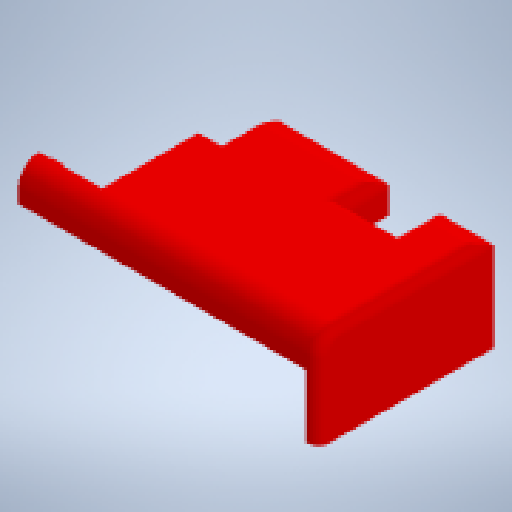
# Autodesk Inventor part: hand_finger_cover
Saved by Autodesk Inventor 2024.1 (Build 281209000, 209)
## iProperties
Created: 2025-03-27
Part Number: hand_finger_cover
Material: 一般
Document SubType Name: Modeling
Designer: hibik
Density: 1 g/cm^3
Appearance: 既定
Author: hibik
Autodesk Inventor part; units mm, degrees
ref_plane "YZ Plane" through (0, 0, 0) normal (1, 0, 0) x (0, 1, 0)
ref_plane "XZ Plane" through (0, 0, 0) normal (0, 1, 0) x (-1, 0, 0)
ref_plane "XY Plane" through (0, 0, 0) normal (0, 0, 1) x (1, 0, 0)
sketch "スケッチ1" plane through (0, 0, 0) normal (1, 0, 0) x (0, 1, 0)
  line L0 (0, 0) -> (22.8, 0)
  line L1 (22.8, 0) -> (22.8, 41.3)
  line L2 (22.8, 41.3) -> (0, 41.3)
  line L3 (0, 41.3) -> (0, 0)
  arc A0 (2, -7.1682) -> (22.8, 4.7165) centre (7.1, 8.05) ccw projected
  line L4 (22.8, 36.2) -> (22.8, 4.7165) projected
  line L5 (22.8, 36.2) -> (12.6, 36.2) projected
  line L6 (12.6, 36.2) -> (12.6, 28.2) projected
  line L7 (14.2, 28.2) -> (12.6, 28.2) projected
  line L8 (14.2, 28.2) -> (14.2, 32.2) projected
  line L9 (14.2, 32.2) -> (20.8, 32.2) projected
  line L10 (20.8, 32.2) -> (20.8, 8.3) projected
  line L11 (14.2, 8.3) -> (20.8, 8.3) projected
  line L12 (14.2, 4.7954) -> (14.2, 8.3) projected
  line L13 (14.2, 0) -> (14.2, 4.7954) projected
  line L14 (2, 0) -> (14.2, 0) projected
  line L15 (2, 0) -> (2, -7.1682) projected
  line L16 (12.6, 42.3) -> (14.6, 42.3) projected
  dimension "d2" = 1
  constraints: 8 end point, 2 parallel, 1 collinear, 1 horizontal, 1 perpendicular
  measures "d2" distance between parallel lines of L2 L16
extrude "押し出し1" add sketch "スケッチ1" along normal blind 1 contours L3 L2 L1 L5 L6 L7 L8 L9 L10 L11 L12 L13 L0 | L13 L12 L11 L10 L9 L8 L7 L6 L5 L1 A0 L0 | A0 L1 L0
sketch "スケッチ2" plane through (0, 0, 0) normal (-1, 0, 0) x (0, 0, 1)
  line L0 (24.3426, 2) -> (36.2, 2)
  line L1 (36.2, 0) -> (36.2, 2)
  arc A0 (25.6, 7.1) -> (20.1, 12.6) centre (20.1, 7.1) ccw
  line L2 (25.6, 7.1) -> (25.6, 5.5)
  arc A1 (24.3426, 2) -> (25.6, 5.5) centre (20.1, 5.5) ccw
  line L3 (0, 12.6) -> (20.1, 12.6)
  line L4 (0, 22.8) -> (41.3, 22.8)
  line L5 (0, 0) -> (0, 22.8)
  line L6 (41.3, 0) -> (0, 0)
  line L7 (41.3, 22.8) -> (41.3, 0)
  line L8 (0, 12.8) -> (20.1, 12.8)
  arc A2 (25.8, 7.1) -> (20.1, 12.8) centre (20.1, 7.1) ccw
  arc A3 (24.7476, 2.2) -> (25.8, 5.5) centre (20.1, 5.5) ccw
  line L9 (25.8, 5.5) -> (25.8, 7.1)
  line L10 (24.7476, 2.2) -> (36.4, 2.2)
  line L11 (36.4, 2.2) -> (36.4, 0)
  line L12 (41.3, 0) -> (0, 0)
  line L13 (0, 0) -> (0, 22.8)
extrude "押し出し2" add sketch "スケッチ2" along normal blind 2 contours L11 L10 A3 L9 A2 L8 L5 L4 L7 L6
sketch "スケッチ3" plane through (-2, 0, 0) normal (-1, 0, 0) x (0, 0, 1)
  line L0 (28.2, 12.6) -> (50.1, 12.6) projected
  line L1 (0, 14.2) -> (4.55, 14.2) projected
  line L2 (41.3, 0) -> (41.3, 22.8) projected
  line L3 (41.3, 22.8) -> (0, 22.8) projected
  line L4 (0, 22.8) -> (0, 12.8) projected
  line L5 (0, 12.8) -> (20.1, 12.8) projected
  arc A0 (25.8, 7.1) -> (20.1, 12.8) centre (20.1, 7.1) ccw projected
  line L6 (25.8, 7.1) -> (25.8, 5.5) projected
  arc A1 (24.7476, 2.2) -> (25.8, 5.5) centre (20.1, 5.5) ccw projected
  line L7 (24.7476, 2.2) -> (36.4, 2.2) projected
  line L8 (36.4, 2.2) -> (36.4, 0) projected
  line L9 (36.4, 0) -> (41.3, 0) projected
  line L10 (41.3, 0) -> (41.3, 22.8) projected
  line L11 (0, 14.7) -> (41.3, 14.7)
  point P0 (0, 0)
  dimension "d9" = 0.5
  constraints: 2 end point, 2 point on line, 1 perpendicular
  measures "d9" distance between parallel lines of L11 L1
extrude "押し出し3" add sketch "スケッチ3" along normal blind 47.4 contours L11 L4 L3 L2
sketch "スケッチ4" plane through (-49.4, 0, 0) normal (-1, 0, 0) x (0, 0, 1)
  line L0 (11.075, 12.3395) -> (13.693, 16.874) projected
  line L1 (13.693, 16.874) -> (13.693, 22.8)
  line L2 (41.3, 22.8) -> (0, 22.8) projected
  line L3 (0, 22.8) -> (0, 14.7) projected
  line L4 (0, 14.7) -> (41.3, 14.7) projected
  line L5 (41.3, 14.7) -> (41.3, 22.8) projected
  line L6 (41.3, 22.8) -> (0, 22.8) projected
  arc A0 (4.7165, 22.8) -> (-7.1682, 2) centre (8.05, 7.1) ccw projected
  line L7 (36.2, 22.8) -> (4.7165, 22.8) projected
  line L8 (36.2, 22.8) -> (36.2, 12.6) projected
  line L9 (36.2, 12.6) -> (28.2, 12.6) projected
  line L10 (28.2, 14.2) -> (28.2, 12.6) projected
  line L11 (28.2, 14.2) -> (32.2, 14.2) projected
  line L12 (32.2, 14.2) -> (32.2, 20.8) projected
  line L13 (32.2, 20.8) -> (8.3, 20.8) projected
  line L14 (8.3, 14.2) -> (8.3, 20.8) projected
  line L15 (4.7954, 14.2) -> (8.3, 14.2) projected
  line L16 (0, 14.2) -> (4.7954, 14.2) projected
  line L17 (0, 2) -> (0, 14.2) projected
  line L18 (0, 2) -> (-7.1682, 2) projected
  point P0 (0, 0)
  point P1 (13.693, 20.8)
  point P2 (32.2, 14.7)
  constraints: 2 end point, 1 perpendicular, 1 point on line
ref_plane "作業平面1" through (-54.9, 2, -8) normal (1, 0, 0) x (0, 1, 0)
extrude "押し出し4" add sketch "スケッチ4" along normal up to surface (5.5 mm away) contours L12 L13 L1 L2 L8 L4 | L8 L2 L5 L4
sketch "スケッチ5" plane through (-54.9, 14.7, 41.3) normal (-1, 0, 0) x (0, 0, 1)
  line L0 (-27.607, 6.1) -> (-9.1, 6.1) projected
  line L1 (-9.1, 6.1) -> (-9.1, 0) projected
  line L2 (-9.1, 0) -> (0, 0) projected
  line L3 (0, 0) -> (0, 8.1) projected
  line L4 (0, 8.1) -> (-27.607, 8.1) projected
  line L5 (-27.607, 8.1) -> (-27.607, 6.1) projected
  line L6 (-5.1, -12.7) -> (-5.1, 0.5) projected
  line L7 (0, 0) -> (-41.3, 0) projected
  line L8 (-4.9, 0) -> (-4.9, 8.1)
  point P0 (-41.3, -14.7)
  point P1 (-4.9, 0)
  dimension "d14" = 0.2
  constraints: 2 end point, 1 point on line, 1 vertical, 2 other
  measures "d14" distance between parallel lines of L6 L8
ref_plane "作業平面2" through (-69.8, 2, -8) normal (-1, 0, 0) x (0, 0, 1)
extrude "押し出し5" add sketch "スケッチ5" along normal up to surface (14.9 mm away) contours L4 L3 L2 L8
sketch "スケッチ6" plane through (-49.4, 0, 0) normal (-1, 0, 0) x (0, 0, 1)
  line L0 (13.693, 20.8) -> (13.693, 22.8) projected
  line L1 (13.693, 22.8) -> (0, 22.8) projected
  line L2 (0, 22.8) -> (0, 14.7) projected
  line L3 (0, 14.7) -> (32.2, 14.7) projected
  line L4 (32.2, 14.7) -> (32.2, 20.8) projected
  line L5 (32.2, 20.8) -> (13.693, 20.8) projected
  line L6 (13.693, 20.8) -> (13.693, 14.7)
  point P0 (0, 0)
  constraints: 2 end point, 1 perpendicular, 1 point on line
extrude "押し出し6" cut sketch "スケッチ6" against normal up to surface (47.4 mm away) contours L5 L4 L3 L6
fillet "フィレット1" radius 5 1 edges at (-34.4, 22.8, 41.3)
fillet "フィレット2" radius 2.5 3 edges at (1, 22.8, 18.15) (1, 21.3355, 39.8355) (1, 8.9, 41.3)
sketch "スケッチ7" plane through (-49.4, 0, 0) normal (-1, 0, 0) x (0, 0, 1)
  arc A0 (4.7165, 22.8) -> (-7.1682, 2) centre (8.05, 7.1) ccw projected
  line L0 (13.693, 22.8) -> (0, 22.8) projected
  arc A1 (4.7165, 22.8) -> (-7.1682, 2) centre (8.05, 7.1) ccw projected
  line L1 (0, 22.8) -> (0, 14.7) projected
  point P0 (0, 0)
  point P1 (0, 20.9852)
extrude "押し出し7" cut sketch "スケッチ7" against normal through all
sketch "スケッチ8" plane through (0, 0, 0) normal (0, 0, -1) x (-1, 0, 0)
  line L0 (23.7, 13.1) -> (23.7, 1.1) projected
  line L1 (2, 14.7) -> (49.4, 14.7) projected
  line L2 (1.5, 22.8) -> (49.4, 22.8) projected
  line L3 (2, 14.7) -> (69.8, 14.7) projected
  line L4 (23.7, 14.7) -> (11.7, 14.7)
  line L5 (11.7, 14.7) -> (11.7, 22.8)
  line L6 (11.7, 22.8) -> (23.7, 22.8)
  line L7 (23.7, 22.8) -> (23.7, 14.7)
  point P0 (0, 0)
  point P1 (11.7, 14.7)
  dimension "d23" = 12
  constraints: 8 end point, 2 collinear, 2 parallel, 1 horizontal, 1 perpendicular, 1 point on line
  measures "d23" distance between parallel lines of L7 L5
extrude "押し出し8" cut sketch "スケッチ8" against normal blind 10
fillet "フィレット3" radius 3 3 edges at (-23.7, 22.8, 7.3582) (-11.7, 22.8, 7.3582) (-17.7, 22.8, 10)
sketch "スケッチ9" plane through (-69.8, 14.7, 36.4) normal (-1, 0, 0) x (0, 0, 1)
  line L0 (-0.2, 0.5) -> (-3.2, 0.5) projected
  line L1 (-0.2, 5.5) -> (-0.2, 0.5) projected
  line L2 (-3.2, 5.5) -> (-0.2, 5.5) projected
  line L3 (-3.2, 0.5) -> (-3.2, 5.5) projected
  line L4 (-3, 5.4) -> (0, 5.4)
  line L5 (0, 5.4) -> (0, 0.6)
  line L6 (0, 0.6) -> (-3, 0.6)
  line L7 (-3, 0.6) -> (-3, 5.4)
  arc A0 (4.9, 3.1) -> (0, 8.099) centre (-0.1, 3.1) ccw projected
  line L8 (0, 0) -> (0, 8.099) projected
  line L9 (4.9, 0) -> (0, 0) projected
  line L10 (4.9, 3.1) -> (4.9, 0) projected
  line L11 (0, 0) -> (0, 8.099) projected
  point P0 (-36.4, -14.7)
  point P1 (-0.2, 3)
  point P2 (-3, 3)
  dimension "d27" = 4.8
  constraints: 8 end point, 3 parallel, 2 midpoint, 1 collinear, 1 horizontal, 1 horizontal alignment, 1 perpendicular
  measures "d27" distance of L6.end L4.start
extrude "押し出し9" add sketch "スケッチ9" against normal blind 2.8 contours L6 L7 L4 L1 | L1 L4 L5 L6
sketch "スケッチ10" plane through (1, 0, 0) normal (1, 0, 0) x (0, 0, -1)
  circle A0 centre (-7.05, 5.504) radius 1.6
  arc A1 (-4.65, 5.508) -> (-6.95, 8) centre (-7.15, 5.508) ccw projected
  arc A2 (-6.95, 8) -> (-9.45, 5.5) centre (-6.95, 5.5) ccw projected
  line L0 (-7.15, 5.508) -> (-6.95, 5.5)
  point P0 (0, 0)
  dimension "d30" = 3.2
  constraints: 2 end point, 1 centre point, 1 coincident, 1 midpoint
  measures "d30" diameter of A0
extrude "押し出し10" cut sketch "スケッチ10" against normal through all
equation "\"d4\" = d3"
equation "\"d5\" = d4"
equation "\"d6\" = d5"
equation "\"d3\" = 0.2"
